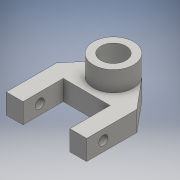
# Autodesk Inventor part: con rod guide
Saved by Autodesk Inventor 2016 (Build 200138000, 138)
## iProperties
Created: 2017-08-15
Part Number: con rod guide
Material: Generic
Document SubType Name: Modeling
Designer: zimirken
Density: 1 g/cm^3
Appearance: Default
Author: zimirken
Autodesk Inventor part; units mm, degrees
ref_plane "YZ Plane" through (0, 0, 0) normal (1, 0, 0) x (0, 1, 0)
ref_plane "XZ Plane" through (0, 0, 0) normal (0, 1, 0) x (-1, 0, 0)
ref_plane "XY Plane" through (0, 0, 0) normal (0, 0, 1) x (1, 0, 0)
sketch "Sketch1" plane through (0, 0, 0) normal (0, 0, 1) x (1, 0, 0)
  line L0 (-14, -16) -> (14, -16)
  line L1 (14, -16) -> (14, -40)
  line L2 (14, -40) -> (24, -40)
  line L3 (24, -40) -> (24, -10)
  line L4 (24, -10) -> (9.2068, 7.6964)
  line L5 (-14, -16) -> (-14, -40)
  line L6 (-14, -40) -> (-24, -40)
  line L7 (-24, -40) -> (-24, -10)
  line L8 (-24, -10) -> (-9.2068, 7.6964)
  arc A0 (9.2068, 7.6964) -> (-9.2068, 7.6964) centre (0, 0) ccw
  circle A1 centre (0, 0) radius 7.5
  point P0 (0, -16)
  dimension "d0" = 28
  dimension "d1" = 10
  dimension "d2" = 24
  dimension "d3" = 40
  dimension "d4" = 30
  dimension "d5" = 15
  dimension "d6" = 12
  constraints: 18 end point, 5 perpendicular, 4 equal length, 2 centre point, 2 coincident, 2 point on circle, 1 horizontal, 1 midpoint, 1 tangent, 1 vertical, 1 vertical alignment
  measures "d0" distance between parallel lines of L1 L5
  measures "d1" distance of L1.end L2.end
  measures "d2" distance between parallel lines of L6 L0
  measures "d3" distance from line of L6 point (0, 0)
  measures "d4" distance of L6.end L7.end
  measures "d5" diameter of A1
  measures "d6" radius of A0
extrude "Extrusion1" add sketch "Sketch1" along normal blind 12
sketch "Sketch2" plane through (24, -40, 0) normal (1, 0, 0) x (0, 0, -1)
  line L0 (0, 0) -> (0, 30) construction
  line L1 (0, 30) -> (-12, 30) construction
  line L2 (-12, 0) -> (-12, 30) construction
  line L3 (0, 0) -> (-12, 0) construction
  line L4 (0, 0) -> (-12, 0) construction
  line L5 (-6, 0) -> (-6, 10) construction
  circle A0 centre (-6, 10) radius 2.75
  point P0 (0, 40)
  dimension "d9" = 10
  dimension "d10" = 5.5
  constraints: 2 end point, 1 centre point, 1 coincident, 1 midpoint, 1 vertical
  measures "d9" distance of L5.start L5.end
  measures "d10" diameter of A0
extrude "Extrusion2" cut sketch "Sketch2" against normal through all
sketch "Sketch3" plane through (0, 0, 12) normal (0, 0, 1) x (1, 0, 0)
  circle A0 centre (0, 0) radius 7.5 projected
  arc A1 (9.2068, 7.6964) -> (-9.2068, 7.6964) centre (0, 0) ccw construction
  circle A2 centre (0, 0) radius 12
  constraints: 1 centre point, 1 coincident, 1 concentric
extrude "Extrusion3" add sketch "Sketch3" along normal blind 12
body "Solid1"
